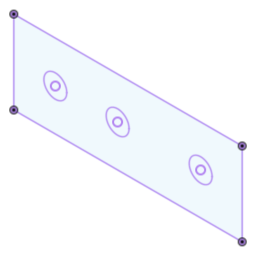
pulley_mount (Autodesk Fusion 360 design; units mm, degrees)
Autodesk Fusion 360 part; units mm, degrees
sketch "Sketch1" plane through (0, 0, 0) normal (0, 0, 1) x (1, 0, 0)
  line L0 (10, 15) -> (65, 15)
  line L1 (65, 15) -> (65, 35)
  line L2 (65, 35) -> (10, 35)
  line L3 (10, 35) -> (10, 15)
  line L4 (10, 15) -> (65, 35) construction
  line L5 (65, 15) -> (10, 35) construction
  line L6 (20, 45) -> (20, 5) construction
  line L7 (35, 5) -> (35, 45) construction
  line L8 (55, 45) -> (55, 5) construction
  line L9 (2.8161, 25) -> (72.658, 25) construction
  circle A0 centre (20, 25) radius 2.75
  circle A1 centre (35, 25) radius 2.75
  circle A2 centre (55, 25) radius 2.75
  point P0 (37.5, 25)
  dimension "d1" = 20
  dimension "d2" = 55
  dimension "d3" = 10
  dimension "d4" = 25
  dimension "d5" = 45
  dimension "d6" = 5.5
  dimension "d7" = 5.5
  dimension "d8" = 5.5
  constraint horizontal L0
  constraint perpendicular L0 L1
  constraint parallel L0 L2
  constraint parallel L1 L3
  constraint coincident L4 P0
  constraint coincident L5 P0
  constraint perpendicular L0 L6
  constraint perpendicular L2 L7
  constraint parallel L7 L8
  constraint perpendicular L1 L9
  constraint midpoint L6 A0.centre
  constraint midpoint L7 A1.centre
  constraint midpoint L8 A2.centre
  measures "d1" distance of L0.start L2.end
  measures "d2" distance of L1.end L2.end
  measures "d3" distance of L3 L6
  measures "d4" distance of L3 L7
  measures "d5" distance of L3 L8
  measures "d6" diameter of A0
  measures "d7" diameter of A1
  measures "d8" diameter of A2
extrude "Extrude1" add sketch "Sketch1" along normal blind 6
sketch "Sketch3" plane through (0, 0, 6) normal (0, 0, 1) x (1, 0, 0)
  circle A0 centre (20, 25) radius 2.75
  circle A1 centre (55, 25) radius 2.75
  circle A2 centre (35, 25) radius 2.75
  line L0 (10, 35) -> (10, 15)
  line L1 (10, 15) -> (65, 15)
  line L2 (65, 15) -> (65, 35)
  line L3 (65, 35) -> (10, 35)
  circle A3 centre (35, 25) radius 2.75
  circle A4 centre (55, 25) radius 2.75
  circle A5 centre (20, 25) radius 2.75
  line L4 (65, 35) -> (10, 35)
  line L5 (65, 15) -> (65, 35)
  line L6 (10, 15) -> (65, 15)
  line L7 (10, 35) -> (10, 15)
hidden bodies 1
